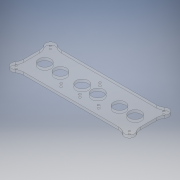
# Autodesk Inventor part: Top
Saved by Autodesk Inventor 2017 (Build 210142000, 142)
## iProperties
Created: 2017-04-15
Part Number: Top
Material: Generic
Document SubType Name: Modeling
Designer: jeffkub
Density: 1 g/cm^3
Appearance: Polycarbonate - Clear
Author: jeffkub
Autodesk Inventor part; units mm, degrees
ref_plane "YZ Plane" through (0, 0, 0) normal (1, 0, 0) x (0, 1, 0)
ref_plane "XZ Plane" through (0, 0, 0) normal (0, 1, 0) x (-1, 0, 0)
ref_plane "XY Plane" through (0, 0, 0) normal (0, 0, 1) x (1, 0, 0)
sketch "Sketch2" plane through (0, 0, 0) normal (0, 1, 0) x (-1, 0, 0)
  line L0 (-94, 28.5) -> (94, 28.5) construction
  line L1 (94, 28.5) -> (94, -28.5) construction
  line L2 (94, -28.5) -> (-94, -28.5) construction
  line L3 (-94, -28.5) -> (-94, 28.5) construction
  line L4 (-94, 28.5) -> (94, -28.5) construction
  line L5 (94, 28.5) -> (-94, -28.5) construction
  line L6 (78.6703, -31.5) -> (-78.6703, -31.5)
  line L7 (-97, -13.1703) -> (-97, 13.1703)
  line L8 (-78.6703, 31.5) -> (78.6703, 31.5)
  line L9 (97, 13.1703) -> (97, -13.1703)
  arc A0 (89.2832, -34.9615) -> (100.4615, -23.7832) centre (94, -28.5) ccw
  arc A1 (100.4615, 23.7832) -> (89.2832, 34.9615) centre (94, 28.5) ccw
  arc A2 (-89.2832, 34.9615) -> (-100.4615, 23.7832) centre (-94, 28.5) ccw
  arc A3 (-100.4615, -23.7832) -> (-89.2832, -34.9615) centre (-94, -28.5) ccw
  arc A4 (89.2832, -34.9615) -> (78.6703, -31.5) centre (78.6703, -49.5) ccw
  arc A5 (97, -13.1703) -> (100.4615, -23.7832) centre (115, -13.1703) ccw
  arc A6 (100.4615, 23.7832) -> (97, 13.1703) centre (115, 13.1703) ccw
  arc A7 (78.6703, 31.5) -> (89.2832, 34.9615) centre (78.6703, 49.5) ccw
  arc A8 (-89.2832, 34.9615) -> (-78.6703, 31.5) centre (-78.6703, 49.5) ccw
  arc A9 (-97, 13.1703) -> (-100.4615, 23.7832) centre (-115, 13.1703) ccw
  arc A10 (-100.4615, -23.7832) -> (-97, -13.1703) centre (-115, -13.1703) ccw
  arc A11 (-78.6703, -31.5) -> (-89.2832, -34.9615) centre (-78.6703, -49.5) ccw
  circle A12 centre (94, -28.5) radius 1.6
  circle A13 centre (94, 28.5) radius 1.6
  circle A14 centre (-94, -28.5) radius 1.6
  circle A15 centre (-94, 28.5) radius 1.6
  circle A16 centre (94, -28.5) radius 3 construction
  circle A17 centre (94, 28.5) radius 3 construction
  circle A18 centre (-94, 28.5) radius 3 construction
  circle A19 centre (-94, -28.5) radius 3 construction
  point P0 (0, 0)
  point P1 (86.5838, -31.5)
  point P2 (-86.5838, -31.5)
  point P3 (-97, -21.0838)
  point P4 (-97, 21.0838)
  point P5 (-86.5838, 31.5)
  point P6 (86.5838, 31.5)
  point P7 (97, 21.0838)
  point P8 (97, -21.0838)
  dimension "d6" = 3
  dimension "d7" = 3
  dimension "d8" = 3
  dimension "d9" = 3
  dimension "d10" = 8
  dimension "d11" = 18
  dimension "d14" = 3.2
  dimension "d15" = 63
  dimension "d16" = 194
  dimension "d17" = 6
  constraints: 32 point on circle, 20 centre point, 20 end point, 16 equal radius, 16 tangent, 12 coincident, 8 point on line, 3 horizontal, 3 parallel, 2 midpoint, 1 perpendicular, 1 vertical
  measures "d6" distance between parallel lines of L2 L6
  measures "d7" distance between parallel lines of L8 L0
  measures "d8" distance between parallel lines of L1 L9
  measures "d9" distance between parallel lines of L3 L7
  measures "d10" radius of A0
  measures "d11" radius of A4
  measures "d14" diameter of A12
  measures "d15" distance between parallel lines of L8 L6
  measures "d16" distance between parallel lines of L7 L9
  measures "d17" diameter of A16
extrude "Extrusion1" add sketch "Sketch2" along normal blind 4.5
sketch "Sketch4" plane through (0, 4.5, 0) normal (0, 1, 0) x (1, 0, 0)
  circle A0 centre (-13, 0) radius 10
  circle A1 centre (13, 0) radius 10
  circle A2 centre (-75, 0) radius 10
  circle A3 centre (-49, 0) radius 10
  circle A4 centre (49, 0) radius 10
  circle A5 centre (75, 0) radius 10
  circle A6 centre (-31, -16.75) radius 1.9
  circle A7 centre (0, -16.75) radius 1.9
  circle A8 centre (31, -16.75) radius 1.9
  circle A9 centre (0, 16.75) radius 1.9
  point P0 (0, 0)
  dimension "d23" = 26
  dimension "d24" = 13
  dimension "d25" = 20
  dimension "d26" = 36
  dimension "d27" = 26
  dimension "d28" = 36
  dimension "d29" = 26
  dimension "d32" = 31
  dimension "d33" = 31
  dimension "d34" = 16.75
  dimension "d35" = 16.75
  dimension "d36" = 3.8
  constraints: 10 centre point, 8 equal radius, 8 horizontal alignment, 2 vertical alignment
  measures "d23" distance of A1.centre A0.centre
  measures "d24" distance of point (0, 0) A1.centre
  measures "d25" diameter of A1
  measures "d26" distance of A0.centre A3.centre
  measures "d27" distance of A2.centre A3.centre
  measures "d28" distance of A4.centre A1.centre
  measures "d29" distance of A5.centre A4.centre
  measures "d32" distance of A6.centre A7.centre
  measures "d33" distance of A8.centre A7.centre
  measures "d34" distance of A7.centre point (0, 0)
  measures "d35" distance of point (0, 0) A9.centre
  measures "d36" diameter of A7
extrude "Extrusion3" cut sketch "Sketch4" against normal through all
equation "\"d7\" = d6"
equation "\"d8\" = d6"
equation "\"d9\" = d8"
equation "\"d24\" = 0.5 * d23"
equation "\"d27\" = d23"
equation "\"d28\" = d26"
equation "\"d29\" = d23"
equation "\"d33\" = d32"
equation "\"d35\" = d34"
body "Solid1"
